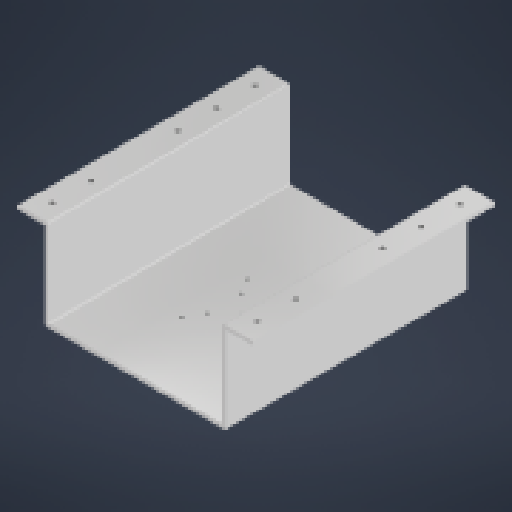
# Autodesk Inventor part: Lower joint housing
Saved by Autodesk Inventor 2026.3 (Build 303398000, 398)
## iProperties
Created: 2026-07-26
Part Number: Lower joint housing
Material: Generic
Document SubType Name: Sheet Metal
Designer: matot
Density: 1 g/cm^3
Sheet Metal Rule: Default_mm
Appearance: Default
Author: matot
Autodesk Inventor part; units mm, degrees
ref_plane "YZ Plane" through (0, 0, 0) normal (1, 0, 0) x (0, 1, 0)
ref_plane "XZ Plane" through (0, 0, 0) normal (0, 1, 0) x (-1, 0, 0)
ref_plane "XY Plane" through (0, 0, 0) normal (0, 0, 1) x (1, 0, 0)
sketch "Sketch1" plane through (0, 0, 0) normal (0, 0, 1) x (1, 0, 0)
  line L0 (98, 0) -> (98, -90)
  line L1 (98, -90) -> (-90, -90)
  line L2 (-90, -90) -> (-90, 0)
  line L3 (126, 4) -> (126, 0)
  line L4 (126, 0) -> (-118, 0)
  line L5 (-118, 0) -> (-118, 4)
  line L6 (-86, 4) -> (94, 4)
  line L7 (94, 4) -> (94, -86)
  line L8 (94, -86) -> (-86, -86)
  line L9 (-86, -86) -> (-86, 4)
  line L10 (-90, 0) -> (-86, 0)
  line L11 (94, 0) -> (98, 0)
  line L12 (-118, 4) -> (-86, 4)
  line L13 (94, 4) -> (126, 4)
  point P0 (0, 0)
  point P1 (6, -4)
  point P2 (126, 2)
  point P3 (98, 0)
  dimension "d0" = 188
  dimension "d1" = 90
  dimension "d3" = 90
  dimension "d4" = 244
  dimension "d5" = 120
  dimension "d8" = 90
  dimension "d9" = 180
  dimension "d10" = 4
  dimension "d13" = 0
  dimension "d14" = 4
  dimension "d90" = 32
  constraints: 28 end point, 8 parallel, 5 horizontal, 5 perpendicular, 2 point on line, 1 midpoint
  measures "d0" distance of L0.end L1.end
  measures "d1" distance of L0.start L0.end
  measures "d3" distance from line of point (0, 0) L2
  measures "d4" distance of L5.end L3.start
  measures "d5" horizontal distance of point (6, -4) point (126, 2)
  measures "d8" distance of L6.end L7.end
  measures "d9" distance of L7.end L8.end
  measures "d10" distance between parallel lines of L0 L7
  measures "d13" distance from line of point (0, 0) L4
  measures "d14" distance between parallel lines of L4 L12
  measures "d90" distance from line of point (126, 2) L7
extrude "Extrusion1" add sketch "Sketch1" along normal blind 250 contours L4 L7 L13 L3 | L0 L1 L2 L4 L9 L8 L7 | L4 L5 L12 L9
fillet "Fillet1" radius 2 4 edges at (-86, -86, 125) (-86, 4, 125) (94, 4, 125) (98, -90, 125)
fillet "Fillet2" radius 2 2 edges at (-90, -90, 125) (94, -86, 125)
sketch "Sketch3" plane through (-84, -86, 250) normal (0, 1, 0) x (1, 0, 0)
  line L0 (-2, 0) -> (-2, 250) projected
  line L1 (176, 0) -> (0, 0) projected
  point P0 (84, 250)
  point P1 (114.75, 74.7)
  point P2 (61.25, 74.7)
  dimension "d28" = 53.5
  dimension "d29" = 63.25
  dimension "d30" = 0
  dimension "d31" = 74.7
  measures "d28" distance of point (61.25, 74.7) point (114.75, 74.7)
  measures "d29" distance from line of L0 point (61.25, 74.7)
  measures "d30" vertical distance of point (114.75, 74.7) point (61.25, 74.7)
  measures "d31" distance from line of L1 point (61.25, 74.7)
hole "Hole2" at (30.75, -86, 175.3) at (-22.75, -86, 175.3) direction (0, -1, 0) diameter 3.4587 end through all thread size "M4x0.5" class "6H" standard "ISO Metric profile"
sketch "Sketch4" plane through (-84, -86, 250) normal (0, 1, 0) x (1, 0, 0)
  circle A0 centre (61.25, 74.7) radius 1.7294 projected
  circle A1 centre (114.75, 74.7) radius 1.7294 projected
  point P0 (84, 250)
  point P1 (114.75, 142.7)
  point P2 (61.25, 142.7)
  dimension "d39" = 53.5
  dimension "d40" = 68
  dimension "d41" = 68
  dimension "d49" = 0
  measures "d39" distance of point (61.25, 142.7) point (114.75, 142.7)
  measures "d40" distance of A0.centre point (61.25, 142.7)
  measures "d41" distance of A1.centre point (114.75, 142.7)
  measures "d49" horizontal distance of point (114.75, 142.7) A1.centre
hole "Hole3" at (30.75, -86, 107.3) at (-22.75, -86, 107.3) direction (0, -1, 0) diameter 3.4587 end through all thread size "M4x0.5" class "6H" standard "ISO Metric profile"
sketch "Sketch5" plane through (-84, -86, 250) normal (0, 1, 0) x (1, 0, 0)
  circle A0 centre (61.25, 74.7) radius 1.7294 projected
  circle A1 centre (114.75, 74.7) radius 1.7294 projected
  circle A2 centre (61.25, 142.7) radius 1.7294 projected
  point P0 (84, 250)
  point P1 (71, 91.2)
  point P2 (71, 126.2)
  point P3 (106, 126.2)
  point P4 (106, 91.2)
  dimension "d50" = 35
  dimension "d51" = 35
  dimension "d52" = 35
  dimension "d53" = 16.5
  dimension "d54" = 16.5
  dimension "d55" = 9.75
  measures "d50" distance of point (71, 126.2) point (71, 91.2)
  measures "d51" distance of point (106, 126.2) point (71, 126.2)
  measures "d52" distance of point (106, 91.2) point (71, 91.2)
  measures "d53" vertical distance of A0.centre point (71, 91.2)
  measures "d54" vertical distance of A1.centre point (106, 91.2)
  measures "d55" horizontal distance of point (71, 126.2) A2.centre
hole "Hole4" at (-13, -86, 158.8) at (-13, -86, 123.8) at (22, -86, 123.8) at (22, -86, 158.8) direction (0, -1, 0) diameter 3.4587 end through all thread size "M4x0.5" class "6H" standard "ISO Metric profile"
sketch "Sketch6" plane through (-84, -86, 250) normal (0, 1, 0) x (1, 0, 0)
  circle A0 centre (71, 126.2) radius 1.7294 projected
  point P0 (84, 250)
  point P1 (88.5, 108.7)
  dimension "d63" = 17.5
  dimension "d64" = 17.5
  measures "d63" horizontal distance of point (88.5, 108.7) A0.centre
  measures "d64" horizontal distance of A0.centre point (88.5, 108.7)
hole "Hole5" at (4.5, -86, 141.3) direction (0, -1, 0) diameter 3 end through all
sketch "Sketch7" plane through (126, 4, 250) normal (0, 1, 0) x (1, 0, 0)
  line L0 (-244, 250) -> (-244, 0) projected
  line L1 (-214, 0) -> (-244, 0) projected
  line L2 (-214, 250) -> (-244, 250) projected
  line L3 (0, 250) -> (0, 0) projected
  line L4 (0, 250) -> (-30, 250) projected
  line L5 (-28, 0) -> (0, 0) projected
  point P0 (-126, 250)
  point P1 (-228, 20)
  point P2 (-228, 60)
  point P3 (-228, 230.025)
  point P4 (-228, 190.025)
  point P5 (-228, 150.025)
  point P6 (-16, 230)
  point P7 (-16, 190)
  point P8 (-16, 150)
  point P9 (-16, 60)
  point P10 (-16, 20)
  point P11 (-229, 250)
  point P12 (-15, 250)
  dimension "d72" = 16
  dimension "d73" = 16
  dimension "d74" = 16
  dimension "d75" = 16
  dimension "d76" = 16
  dimension "d77" = 20
  dimension "d78" = 40
  dimension "d79" = 20
  dimension "d80" = 40
  dimension "d81" = 40
  dimension "d82" = 16
  dimension "d83" = 16
  dimension "d84" = 16
  dimension "d85" = 16
  dimension "d86" = 16
  dimension "d87" = 20
  dimension "d88" = 40
  dimension "d89" = 40
  dimension "d98" = 20
  dimension "d99" = 40
  constraints: 2 midpoint
  measures "d72" distance from line of point (-228, 230.025) L0
  measures "d73" distance from line of point (-228, 190.025) L0
  measures "d74" distance from line of point (-228, 150.025) L0
  measures "d75" distance from line of point (-228, 60) L0
  measures "d76" distance from line of point (-228, 20) L0
  measures "d77" distance from line of L1 point (-228, 20)
  measures "d78" distance of point (-228, 20) point (-228, 60)
  measures "d79" distance of point (-229, 250) point (-228, 230.025)
  measures "d80" distance of point (-228, 190.025) point (-228, 230.025)
  measures "d81" distance of point (-228, 150.025) point (-228, 190.025)
  measures "d82" distance from line of L3 point (-16, 20)
  measures "d83" distance from line of L3 point (-16, 60)
  measures "d84" distance from line of point (-16, 150) L3
  measures "d85" distance from line of L3 point (-16, 190)
  measures "d86" distance from line of L3 point (-16, 230)
  measures "d87" vertical distance of point (-15, 250) point (-16, 230)
  measures "d88" distance of point (-16, 190) point (-16, 230)
  measures "d89" distance of point (-16, 150) point (-16, 190)
  measures "d98" distance from line of L5 point (-16, 20)
  measures "d99" distance of point (-16, 60) point (-16, 20)
hole "Hole6" at (-102, 4, 230) at (-102, 4, 190) at (-102, 4, 19.975) at (-102, 4, 59.975) at (-102, 4, 99.975) at (110, 4, 20) at (110, 4, 60) at (110, 4, 100) at (110, 4, 190) at (110, 4, 230) direction (0, -1, 0) diameter 4.917 end through all thread size "M6x1" class "6H" standard "ISO Metric profile"
equation "\"BendRadius\" = Thickness"
equation "\"BendReliefWidth\" = Thickness"
equation "\"BendReliefDepth\" = 0.5 * Thickness"
equation "\"CornerReliefSize\" = 4 * Thickness"
equation "\"MinimumRemnant\" = 2 * Thickness"
equation "\"TransitionRadius\" = BendRadius"
equation "\"JacobiRadiusSize\" = BendRadius"
equation "\"GapSize\" = Thickness"
equation "\"Thickness\" = 0.5"
body "Solid1"
